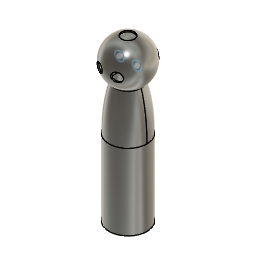
Statue v1 (Autodesk Fusion 360 design; units mm, degrees)
Autodesk Fusion 360 part; units mm, degrees
sketch "Sketch1" plane through (0, 0, 0) normal (0, 1, 0) x (1, 0, 0)
  line L0 (-15, 0) -> (15, 0)
  line L1 (-15, 30) -> (15, 30)
  line L2 (15, 30) -> (15, 0)
  line L3 (-15, 0) -> (-15, 30)
  ellipse E0 centre (0, 0) end of major axis (0, -50) minor radius 15
  line L4 (0, 50) -> (0, -50) construction
  line L5 (-15, 0) -> (15, 0) construction
  line L6 (0, -50) -> (0, 30)
  point P0 (0, -50)
  constraint horizontal L0
  constraint parallel L0 L1
  constraint perpendicular L0 L2
  constraint perpendicular L1 L3
  constraint coincident E0 L4.start
  constraint coincident E0 P0
  constraint coincident E0 L0.start
  constraint coincident E0 L0.end
  constraint coincident E0.centre origin
  constraint perpendicular L0 L4
  constraint coincident L0.end L2.end
  constraint coincident P0 L4.end
  constraint midpoint L1 L6.end
revolve "Revolve1" add sketch "Sketch1" angle 360 about axis through (0, 0, 50) along (0, 0, -1) contours L0 L1 E0 L6 | L0 E0 L6 | L1 L2 E0 picked at (4.7969, 14.702) picked at (3.579, -28.3051) makes body 1
sketch "Sketch2" plane through (0, 0, 0) normal (0, 1, 0) x (1, 0, 0)
  circle A0 centre (75, 0) radius 17.5
  line L0 (75, -17.5) -> (75, 17.5)
  dimension "d4" = 35
  constraint coincident A0 L0.start
  constraint coincident A0 L0.end
  constraint vertical L0
  measures "d4" diameter of A0
revolve "Revolve2" add sketch "Sketch2" angle 360 about axis through (75, 0, 17.5) along (0, 0, -1) separate body contours A0 L0 picked at (84.594, -2.255) makes body 2
copy_body "Body->Comp1" bodies 2 removing the originals makes body 3 in component "Component"
extrude "Extrude1" add 2 faces at (-13.9414, 0, -30) (-3.1999, -0.9573, -30) along direction (0, 0, -1) blind 30 on bodies 1 bodies 1
combine "Combine1" operation add target body 3 tool bodies 1 body 1 seen with x (1, 0, 0) y (0, 1, 0) z (0, 0, 1) at (75, 0, -50) in component "Component"
shell "Shell1" thickness 1 removed faces 1 at (82.0705, 3.0369, -110) on bodies 3 in component "Component"
sketch "Sketch3" plane through (0, 0, 0) normal (0, 0, 1) x (1, 0, 0)
  circle A0 centre (0, 0) radius 5
  dimension "d21" = 10
  constraint coincident A0.centre origin
  measures "d21" diameter of A0
extrude "Extrude1'" cut sketch "Sketch3" along normal blind 120 sketch seen with x (1, 0, 0) y (0, 1, 0) z (0, 0, 1) at (75, 0, -50) bodies 3 in component "Component"
sketch "Sketch4" plane through (0, 0, 0) normal (0, 1, 0) x (1, 0, 0)
  circle A0 centre (-6.7404, -49.3418) radius 3.5
  circle A1 centre (6.9177, -49.4241) radius 3.5
  dimension "d15" = 7
  dimension "d16" = 7
  measures "d15" diameter of A0
  measures "d16" diameter of A1
extrude "Extrude2" cut sketch "Sketch4" along normal mid plane 90 contours A1 sketch seen with x (1, 0, 0) y (0, 1, 0) z (0, 0, 1) at (75, 0, -50) bodies 3 in component "Component"
extrude "Extrude3" cut sketch "Sketch4" along normal mid plane 38 contours A0 sketch seen with x (1, 0, 0) y (0, 1, 0) z (0, 0, 1) at (75, 0, -50) bodies 3 in component "Component"
component "Component" placed x (1, 0, 0) y (0, 1, 0) z (0, 0, 1) at (-75, 0, 50)
